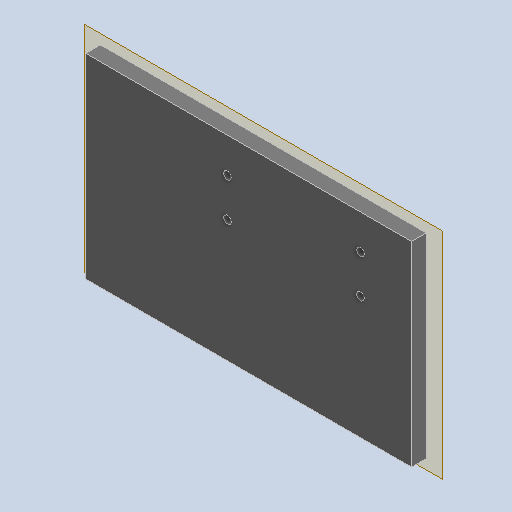
# Autodesk Inventor part: 21
Saved by Autodesk Inventor 2024.3 (Build 283343000, 343)
## iProperties
Created: 2024-09-08
Part Number: 21
Material: 아크릴, 선명
Document SubType Name: Modeling
Designer: 구지현
Density: 1.19 g/cm^3
Appearance: 회색
Author: 구지현
Autodesk Inventor part; units mm, degrees
ref_plane "YZ Plane" through (0, 0, 0) normal (1, 0, 0) x (0, 1, 0)
ref_plane "XZ Plane" through (0, 0, 0) normal (0, 1, 0) x (-1, 0, 0)
ref_plane "XY Plane" through (0, 0, 0) normal (0, 0, 1) x (1, 0, 0)
ref_plane "작업 평면1" through (0, 0, 0) normal (0, 0, 1) x (1, 0, 0)
sketch "스케치1" plane through (0, 0, 0) normal (0, 0, 1) x (1, 0, 0)
  line L0 (66.25, -39.75) -> (66.25, 39.75) projected
  line L1 (66.25, 39.75) -> (-66.25, 39.75) projected
  line L2 (-66.25, 39.75) -> (-66.25, -39.75) projected
  line L3 (-66.25, -39.75) -> (66.25, -39.75) projected
  point P0 (0, 0)
extrude "돌출1" add sketch "스케치1" along normal blind 6
sketch "스케치2" plane through (0, 0, 6) normal (0, 0, 1) x (1, 0, 0)
  line L0 (-5.632, 3.9673) -> (-5.632, 31.5673) projected
  line L1 (-11.632, 3.9673) -> (-11.632, 31.5673) projected
  line L2 (-11.632, 31.5673) -> (-5.632, 31.5673) projected
  line L3 (-5.632, 3.9673) -> (-5.632, 31.5673) projected
  line L4 (-11.632, 3.9673) -> (-5.632, 3.9673) projected
  line L5 (42.469, 4.0673) -> (42.469, 31.6673) projected
  line L6 (42.469, 4.0673) -> (48.469, 4.0673) projected
  line L7 (48.469, 4.0673) -> (48.469, 31.6673) projected
  line L8 (42.469, 31.6673) -> (48.469, 31.6673) projected
  line L9 (-8.632, 31.5673) -> (-8.632, 25.5673)
  circle A0 centre (-8.632, 25.5673) radius 1.55
  line L10 (-8.632, 3.9673) -> (-8.632, 9.9673)
  circle A1 centre (-8.632, 9.9673) radius 1.55
  circle A2 centre (45.469, 10.0673) radius 1.55
  circle A3 centre (45.469, 25.6673) radius 1.55
  point P0 (0, 0)
  dimension "d2" = 6
  dimension "d3" = 3.1
  dimension "d4" = 6
  dimension "d5" = 3.1
  dimension "d6" = 3.1
  dimension "d7" = 3.1
  dimension "d8" = 6
  dimension "d9" = 6
  constraints: 4 centre point, 4 end point, 2 coincident, 2 midpoint, 2 vertical
  measures "d2" distance of L9.start L9.end
  measures "d3" diameter of A0
  measures "d4" distance of L10.start L10.end
  measures "d5" diameter of A1
  measures "d6" diameter of A2
  measures "d7" diameter of A3
  measures "d8" distance from line of A3.centre L8
  measures "d9" distance from line of A2.centre L6
extrude "돌출2" cut sketch "스케치2" against normal blind 6 contours A0 | A1 | A2 | A3
